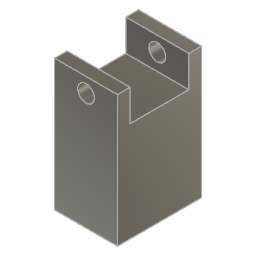
adapter v1 (Autodesk Fusion 360 design; units mm, degrees)
Autodesk Fusion 360 part; units mm, degrees
sketch "Sketch1" plane through (0, 0, 0) normal (0, 0, 1) x (1, 0, 0)
  line L0 (0, 0) -> (15, 0)
  line L1 (15, 0) -> (15, 20)
  line L2 (15, 20) -> (0, 20)
  line L3 (0, 20) -> (0, 0)
  dimension "d1" = 15
  dimension "d2" = 20
  constraint horizontal L0
  constraint vertical L1
  constraint horizontal L2
  constraint vertical L3
  constraint coincident L0.start L3.end
  measures "d1" distance of L0.start L0.end
  measures "d2" distance of L0.end L1.end
extrude "Extrude1" add sketch "Sketch1" along normal blind 1.3
sketch "Sketch3" plane through (0, 0, 1.3) normal (0, 0, 1) x (-1, 0, 0)
  line L0 (0, -20) -> (0, 0)
  line L1 (0, 0) -> (-15, 0)
  line L2 (-15, 0) -> (-15, -20)
  line L3 (-15, -20) -> (0, -20)
  line L4 (-8.65, -4.5) -> (-8.65, -20)
  line L5 (-8.65, -20) -> (-7.5, -20)
  line L6 (-6.35, -4.5) -> (-6.35, -20)
  line L7 (-6.35, -20) -> (-7.5, -20)
  line L8 (-6.35, -3) -> (-8.65, -3)
  line L9 (-6.35, -4.5) -> (-6.35, -3)
  line L10 (-8.65, -4.5) -> (-8.65, -3)
  dimension "d14" = 3
  constraint vertical L4
  constraint horizontal L5
  constraint vertical L6
  constraint horizontal L7
  constraint horizontal L8
  constraint perpendicular L8 L9
  constraint perpendicular L8 L10
  measures "d14" distance of L1 L8
extrude "Extrude2" cut sketch "Sketch3" against normal blind 6 contours L3 L4 L5 L6 L7 L8 L9 L10
sketch "Sketch4" plane through (0, 0, 1.3) normal (0, 0, 1) x (-1, 0, 0)
  line L0 (-6.35, -3) -> (-6.35, -20)
  line L1 (-6.35, -20) -> (0, -20)
  line L2 (0, -20) -> (0, 0)
  line L3 (0, 0) -> (-15, 0)
  line L4 (-15, 0) -> (-15, -20)
  line L5 (-15, -20) -> (-8.65, -20)
  line L6 (-8.65, -20) -> (-8.65, -3)
  line L7 (-8.65, -3) -> (-6.35, -3)
  line L8 (0, 0) -> (-15, 0)
  line L9 (-15, 0) -> (-15, -20)
  line L10 (-15, -20) -> (0, -20)
  line L11 (0, -20) -> (0, 0)
  constraint horizontal L8
  constraint vertical L9
  constraint horizontal L10
  constraint vertical L11
  constraint coincident L4.end L5.start
  constraint coincident L2.end L3.start
extrude "Extrude3" add sketch "Sketch4" along normal blind 30
sketch "Sketch5" plane through (0, 0, 0) normal (-1, 0, 0) x (0, -1, 0)
  line L0 (-20, 0) -> (0, 0)
  line L1 (0, 0) -> (0, 31.3)
  line L2 (0, 31.3) -> (-20, 31.3)
  line L3 (-20, 31.3) -> (-20, 0)
  line L4 (-10, 31.3) -> (-17, 31.3)
  line L5 (-10, 31.3) -> (-3, 31.3)
  line L6 (-17, 31.3) -> (-17, 23.8)
  line L7 (-3, 31.3) -> (-3, 23.8)
  line L8 (-17, 23.8) -> (-3, 23.8)
  dimension "d19" = 7
  dimension "d20" = 7
  dimension "d21" = 7.5
  dimension "d22" = 7.5
  constraint midpoint L2 L4.start
  constraint parallel L2 L4
  constraint parallel L2 L5
  constraint perpendicular L2 L6
  constraint perpendicular L2 L7
  measures "d19" distance of L4.start L4.end
  measures "d20" distance of L4.start L5.end
  measures "d21" distance of L4.end L6.end
  measures "d22" distance of L5.end L7.end
extrude "Extrude4" cut sketch "Sketch5" against normal blind 24 contours L2 L4 L5 L6 L7 L8
sketch "Sketch6" plane through (0, 20, 0) normal (0, 1, 0) x (-1, 0, 0)
  line L0 (-6.35, 1.3) -> (-6.35, 0)
  line L1 (-6.35, 0) -> (0, 0)
  line L2 (0, 0) -> (0, 31.3)
  line L3 (0, 31.3) -> (-15, 31.3)
  line L4 (-15, 31.3) -> (-15, 0)
  line L5 (-15, 0) -> (-8.65, 0)
  line L6 (-8.65, 0) -> (-8.65, 1.3)
  line L7 (-8.65, 1.3) -> (-6.35, 1.3)
  circle A0 centre (-7.5, 27.8) radius 2
  dimension "d26" = 4
  measures "d26" diameter of A0
extrude "Extrude5" cut sketch "Sketch6" against normal blind 22 contours A0
